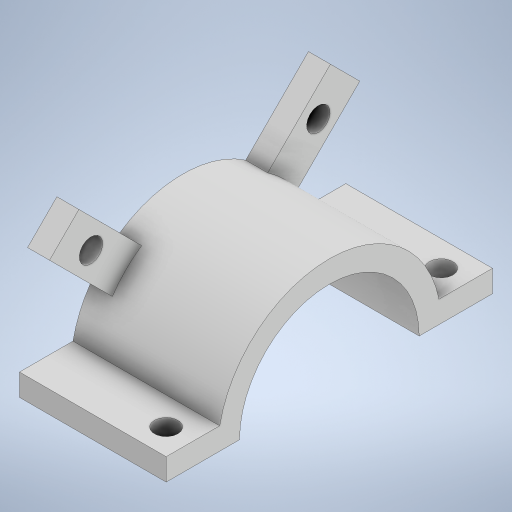
# Autodesk Inventor part: SensorHalterSchale
Saved by Autodesk Inventor 2023 (Build 270158000, 158)
## iProperties
Created: 2024-03-05
Part Number: SensorHalterSchale
Material: Generisch
Document SubType Name: Modeling
Designer: phili
Density: 1 g/cm^3
Appearance: Vorgabe
Author: phili
Autodesk Inventor part; units mm, degrees
ref_plane "YZ Plane" through (0, 0, 0) normal (1, 0, 0) x (0, 1, 0)
ref_plane "XZ Plane" through (0, 0, 0) normal (0, 1, 0) x (-1, 0, 0)
ref_plane "XY Plane" through (0, 0, 0) normal (0, 0, 1) x (1, 0, 0)
sketch "Skizze1" plane through (0, 0, 0) normal (1, 0, 0) x (0, 1, 0)
  arc A0 (0, -12.25) -> (0, 12.25) centre (0, 0) ccw
  arc A1 (0, -15.25) -> (0, 15.25) centre (0, 0) ccw
  line L0 (0, 15.25) -> (0, 12.25)
  line L1 (0, -12.25) -> (0, -15.25)
  dimension "d0" = 12.25
  dimension "d1" = 15.25
  constraints: 4 end point, 4 point on circle, 2 centre point, 2 coincident, 1 collinear, 1 vertical
  measures "d0" radius of A0
  measures "d1" radius of A1
extrude "Extrusion1" add sketch "Skizze1" along normal blind 20
sketch "Skizze7" plane through (0, 0, 0) normal (-1, 0, 0) x (0, 0, 1)
  arc A0 (15.25, 0) -> (-15.25, 0) centre (0, 0) ccw projected
  line L0 (-12.5965, 8.596) -> (-21.1503, 17.1499)
  line L1 (-12.5965, 8.596) -> (-0.4995, 8.596) construction
  line L2 (-21.1503, 17.1499) -> (-17.1502, 21.15)
  line L3 (-17.1502, 21.15) -> (-8.596, 12.5965)
  arc A1 (-8.596, 12.5965) -> (-12.5965, 8.596) centre (0, 0) ccw
  dimension "d40" = 12.097
  dimension "d41" = 135
  dimension "d42" = 8.596
  dimension "d43" = 5.657
  constraints: 8 end point, 5 point on circle, 2 concentric, 1 centre point, 1 equal length, 1 horizontal
  measures "d40" distance of L0.start L0.end
  measures "d41" angle of L1 L0
  measures "d42" vertical distance of L0.start A0.end
  measures "d43" distance of L0.end L2.end
extrude "Extrusion4" add sketch "Skizze7" against normal blind 3
mirror "Spiegeln4" about plane through (0, 0, 0) normal (0, 0, 1) of "Extrusion4"
sketch "Skizze8" plane through (3, 21.15, 17.1502) normal (1, 0, 0) x (0, -0.7070757, -0.7071379)
  line L0 (-0.0002, -5.657) -> (0, 0) projected
  line L1 (29.9122, 24.2528) -> (24.2552, 24.253) projected
  line L2 (24.2552, 24.253) -> (24.2541, 12.156) projected
  line L3 (0, 0) -> (12.097, 0) projected
  point P0 (27.0822, -2.8294)
  point P1 (5.1619, -2.8285)
  point P2 (27.0832, 19.0909)
  point P3 (27.0837, 24.2529)
  dimension "d53" = 5.162
  dimension "d54" = 5.162
  dimension "d55" = 2.8285
  dimension "d56" = 2.8285
  constraints: 1 midpoint
  measures "d53" distance from line of point (5.162, -2.829) L0
  measures "d54" distance of point (27.084, 24.253) point (27.083, 19.091)
  measures "d55" distance from line of L2 point (27.083, 19.091)
  measures "d56" distance from line of L3 point (5.162, -2.829)
hole "Bohrung3" at (3, 15.5, 15.5001) at (3, 15.5, -15.5001) direction (-1, 0, 0) diameter 3.2 end through all
sketch "Skizze9" plane through (0, 0, 0) normal (-1, 0, 0) x (0, 0, 1)
  line L0 (-12.25, 0) -> (-15.25, 0) projected
  line L1 (-15.25, 0) -> (-22.25, 0)
  line L2 (-22.25, 0) -> (-22.25, 3)
  line L3 (-22.25, 3) -> (-14.952, 3)
  arc A0 (-12.5965, 8.596) -> (-15.25, 0) centre (0, 0) ccw projected
  arc A1 (-14.952, 3) -> (-15.25, 0) centre (0, 0) ccw
  dimension "d57" = 7
  dimension "d58" = 3
  constraints: 6 end point, 3 point on circle, 2 perpendicular, 1 centre point, 1 concentric, 1 horizontal
  measures "d57" distance of L0.end L1.end
  measures "d58" distance of L1.end L2.end
extrude "Extrusion5" add sketch "Skizze9" against normal blind 20
sketch "Skizze10" plane through (0, 0, -12.25) normal (0, -1, 0) x (1, 0, 0)
  line L0 (20, 0) -> (20, -10) projected
  line L1 (0, -10) -> (20, -10) projected
  point P0 (0, 12.25)
  point P1 (16.5, -6.5)
  dimension "d68" = 3.5
  dimension "d69" = 3.5
  measures "d68" distance from line of L0 point (16.5, -6.5)
  measures "d69" distance from line of point (16.5, -6.5) L1
hole "Bohrung4" at (16.5, 0, -18.75) direction (0, 1, 0) diameter 3.2 end through all
mirror "Spiegeln5" about plane through (0, 0, 0) normal (0, 0, 1) of "Extrusion5", "Bohrung4"
